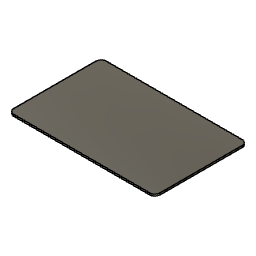
ID Card_ (Autodesk Fusion 360 design; units mm, degrees)
Autodesk Fusion 360 part; units mm, degrees
sketch "Sketch1" plane through (0, 0, 0) normal (0, 0, 1) x (1, 0, 0)
  line L0 (-3, 0) -> (-82.5, 0)
  line L1 (-85.5, 3) -> (-85.5, 51)
  line L2 (-82.5, 54) -> (-3, 54)
  line L3 (0, 51) -> (0, 3)
  arc A0 (0, 51) -> (-3, 54) centre (-3, 51) ccw
  arc A1 (-82.5, 54) -> (-85.5, 51) centre (-82.5, 51) ccw
  arc A2 (-85.5, 3) -> (-82.5, 0) centre (-82.5, 3) ccw
  arc A3 (-3, 0) -> (0, 3) centre (-3, 3) ccw
  point P0 (-85.5, 0)
  point P1 (0, 54)
  dimension "d1" = 85.5
  dimension "d2" = 54
  dimension "d3" = 3
  dimension "d4" = 3
  dimension "d5" = 3
  dimension "d6" = 3
  constraint horizontal L0
  constraint vertical L1
  constraint horizontal L2
  constraint vertical L3
  constraint coincident P1 L2
  constraint coincident P1 L3
  constraint tangent L2 A0
  constraint tangent L3 A0
  constraint tangent L1 A1
  constraint tangent L2 A1
  constraint coincident P0 L0
  constraint coincident P0 L1
  constraint tangent L0 A2
  constraint tangent L1 A2
  constraint coincident origin L0
  constraint coincident origin L3
  constraint tangent L0 A3
  constraint tangent L3 A3
  measures "d1" distance of origin P0
  measures "d2" distance of origin P1
  measures "d3" radius of A0
  measures "d4" radius of A1
  measures "d5" radius of A2
  measures "d6" radius of A3
extrude "Extrude1" add sketch "Sketch1" along normal blind 1
